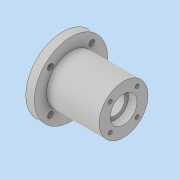
# Autodesk Inventor part: Lagerhalter
Saved by Autodesk Inventor 2018 (Build 220112000, 112)
## iProperties
Created: 2020-05-23
Part Number: Lagerhalter
Material: Generisch
Document SubType Name: Modeling
Designer: marce
Density: 1 g/cm^3
Appearance: Vorgabe
Author: marce
Autodesk Inventor part; units mm, degrees
ref_plane "YZ Plane" through (0, 0, 0) normal (1, 0, 0) x (0, 1, 0)
ref_plane "XZ Plane" through (0, 0, 0) normal (0, 1, 0) x (-1, 0, 0)
ref_plane "XY Plane" through (0, 0, 0) normal (0, 0, 1) x (1, 0, 0)
sketch "Skizze1" plane through (0, 0, 0) normal (0, 0, 1) x (1, 0, 0)
  line L0 (0, 0) -> (0, 17.5)
  line L1 (0, 17.5) -> (5, 17.5)
  line L2 (5, 17.5) -> (5, 20)
  line L3 (5, 20) -> (55, 20)
  line L4 (55, 20) -> (55, 0)
  line L5 (55, 0) -> (0, 0)
  line L6 (0, 11) -> (7, 11)
  line L7 (7, 11) -> (7, 8)
  line L8 (7, 8) -> (48, 8)
  line L9 (48, 8) -> (48, 11)
  line L10 (48, 11) -> (55, 11)
  line L11 (5, 20) -> (12, 20)
  line L12 (12, 20) -> (12, 30)
  line L13 (12, 30) -> (5, 30)
  line L14 (5, 30) -> (5, 20)
  dimension "d1" = 17.5
  dimension "d2" = 5
  dimension "d4" = 50
  dimension "d5" = 8
  dimension "d6" = 11
  dimension "d7" = 7
  dimension "d8" = 7
  dimension "d31" = 20
  dimension "d32" = 7
  dimension "d33" = 30
  constraints: 30 end point, 9 perpendicular, 4 point on line, 2 horizontal, 2 parallel, 1 vertical
  measures "d1" distance of L0.start L0.end
  measures "d2" distance of L0.end L1.end
  measures "d4" distance of L2.end L3.end
  measures "d5" distance between parallel lines of L5 L8
  measures "d6" distance between parallel lines of L5 L6
  measures "d7" distance of L6.start L6.end
  measures "d8" distance of L9.end L10.end
  measures "d31" distance between parallel lines of L5 L3
  measures "d32" distance of L13.end L12.end
  measures "d33" distance between parallel lines of L5 L13
revolve "Umdrehung1" add sketch "Skizze1" angle 360 about axis through (55, 0, 0) along (-1, 0, 0) contours L0 L1 L2 L3 L4 L10 L9 L8 L7 L6 | L14 L13 L12 L3
sketch "Skizze4" plane through (55, 0, 0) normal (1, 0, 0) x (0, 0, -1)
  circle A0 centre (0, 0) radius 15.5
  circle A1 centre (0, 0) radius 11 projected
  circle A2 centre (0, 0) radius 20 projected
  line L0 (10.9602, 10.9602) -> (10.9602, -10.9602)
  line L1 (10.9602, -10.9602) -> (-10.9602, -10.9602)
  line L2 (-10.9602, -10.9602) -> (-10.9602, 10.9602)
  line L3 (-10.9602, 10.9602) -> (10.9602, 10.9602)
  dimension "d20" = 4.5
  dimension "d21" = 4.5
  constraints: 8 end point, 2 coincident, 1 horizontal, 12 other
hole "Bohrung2" at (55, 10.9602, -10.9602) at (55, -10.9602, -10.9602) at (55, -10.9602, 10.9602) at (55, 10.9602, 10.9602) direction (-1, 0, 0) diameter 3.242 depth 10 tip angle 118 thread size "M4x0.7" class "6H" standard "ANSI Metric M Profile"
sketch "Skizze6" plane through (5, 0, 0) normal (-1, 0, 0) x (0, 0, 1)
  circle A0 centre (0, 0) radius 24
  line L0 (-16.9706, 16.9706) -> (16.9706, 16.9706)
  line L1 (16.9706, 16.9706) -> (16.9706, -16.9706)
  line L2 (16.9706, -16.9706) -> (-16.9706, -16.9706)
  line L3 (-16.9706, -16.9706) -> (-16.9706, 16.9706)
  dimension "d34" = 48
  constraints: 8 end point, 2 coincident, 1 vertical, 12 other
hole "Bohrung3" at (5, 16.9706, -16.9706) at (5, -16.9706, -16.9706) at (5, -16.9706, 16.9706) at (5, 16.9706, 16.9706) direction (1, 0, 0) diameter 4.917 depth 17.1 tip angle 118 thread size "M6x1" class "6H" standard "ISO Metric profile"
equation "\"d20\" = d21"
